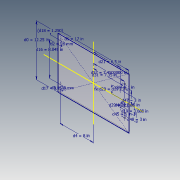
# Autodesk Inventor part: FLUGGER LOADING ACCESS DOOR
Saved by Autodesk Inventor 2020.3 (Build 243373000, 373)
## iProperties
RuleStatus: InUse
AfterDocSave0: file://Part Number Cleaner
Created: 2020-01-19
Material: ACRYLIC, CLEAR
Vendor: HHMI: JRC - ID&F
Document SubType Name: Modeling
Designer: arnoldj
Density: 0.66 g/cm^3
Appearance: Polycarbonate (Clear)
DESIGN DEPARTMENT: HHMI: JRC - ID&F
ALTERED ITEM PART NUMBER: N/A
ALTERED ITEM VENDOR: N/A
ALTERED ITEM DESCRIPTION: N/A
Author: arnoldj
Revision Number: 0
Autodesk Inventor part; units mm, degrees
ref_plane "YZ Plane" through (0, 0, 0) normal (1, 0, 0) x (0, 1, 0)
ref_plane "XZ Plane" through (0, 0, 0) normal (0, 1, 0) x (-1, 0, 0)
ref_plane "XY Plane" through (0, 0, 0) normal (0, 0, 1) x (1, 0, 0)
sketch "Sketch1" plane through (0, 0, 0) normal (0, 0, 1) x (1, 0, 0)
  line L0 (0, 217.805) -> (0, -217.805) projected
  line L1 (-302.26, 0) -> (302.26, 0) projected
  line L2 (215.9, -155.575) -> (-215.9, -155.575)
  line L3 (-215.9, -155.575) -> (-215.9, 155.575)
  line L4 (-215.9, 155.575) -> (215.9, 155.575)
  line L5 (215.9, 155.575) -> (215.9, -155.575)
  line L6 (215.9, -155.575) -> (-215.9, 155.575) construction
  line L7 (-215.9, -155.575) -> (215.9, 155.575) construction
  line L8 (186.69, -13.13) -> (186.69, -35.13) construction
  line L9 (189.23, 88.9) -> (189.23, 63.5) construction
  line L10 (189.23, -63.5) -> (189.23, -88.9) construction
  point P0 (0, 0)
  point P1 (-203.2, 123.818)
  point P2 (-203.2, 95.818)
  point P3 (-203.2, -108.525)
  point P4 (-203.2, -136.525)
  point P5 (165.1, 46.8376)
  point P6 (165.1, -46.8376)
  point P7 (186.69, -24.13)
  point P8 (189.23, -76.2)
  point P9 (189.23, 76.2)
  dimension "d0" = 311.15
  dimension "d1" = 431.8
  dimension "d2" = 28
  dimension "d3" = 28
  dimension "d4" = 203.2
  dimension "d16" = 204.343
  dimension "d17" = 19.05
  dimension "d18" = 31.757
  dimension "d19" = 93.6752
  dimension "d20" = 46.8376
  dimension "d21" = 165.1
  dimension "d29" = 22
  dimension "d31" = 186.69
  dimension "d44" = 25.4
  dimension "d45" = 25.4
  dimension "d46" = 24.13
  dimension "d47" = 76.2
  dimension "d48" = 76.2
  dimension "d57" = 189.23
  constraints: 18 end point, 8 vertical alignment, 5 midpoint, 3 vertical, 2 parallel, 1 horizontal, 1 perpendicular
  measures "d0" distance of L2.end L3.end
  measures "d1" distance of L3.end L4.end
  measures "d2" distance of point (-203.2, 95.818) point (-203.2, 123.818)
  measures "d3" distance of point (-203.2, -108.525) point (-203.2, -136.525)
  measures "d4" distance from line of point (-203.2, -136.525) L0
  measures "d16" distance of point (-203.2, -108.525) point (-203.2, 95.818)
  measures "d17" distance from line of point (-203.2, -136.525) L2
  measures "d18" distance from line of L4 point (-203.2, 123.818)
  measures "d19" distance of point (165.1, -46.838) point (165.1, 46.838)
  measures "d20" distance from line of point (165.1, 46.838) L1
  measures "d21" distance from line of L0 point (165.1, 46.838)
  measures "d29" distance of L8.end L8.start
  measures "d31" distance from line of L0 L8.start
  measures "d44" distance of L9.end L9.start
  measures "d45" distance of L10.start L10.end
  measures "d46" distance from line of L1 point (186.69, -24.13)
  measures "d47" distance from line of L1 point (189.23, 76.2)
  measures "d48" distance from line of point (189.23, -76.2) L1
  measures "d57" distance between parallel lines of L9 L0
extrude "Extrusion1" add sketch "Sketch1" against normal blind 6.35
hole "Hole1-Tap M5" at (-203.2, 123.818, 0) at (-203.2, 95.818, 0) at (-203.2, -108.525, 0) at (-203.2, -136.525, 0) direction (0, 0, -1) diameter 4.064 end through all
hole "Hole2-Tap M5" at (165.1, 46.8376, 0) at (165.1, -46.8376, 0) direction (0, 0, -1) diameter 4.064 end through all
hole "Hole3-Tap M4" at (186.69, -13.13, 0) at (186.69, -35.13, 0) direction (0, 0, -1) diameter 3.1242 end through all
fillet "Fillet1" radius 9.525 4 edges at (-215.9, 155.575, -3.175) (215.9, 155.575, -3.175) (215.9, -155.575, -3.175) (-215.9, -155.575, -3.175)
hole "Hole4 CSINK M4" at (189.23, -88.9, 0) at (189.23, 88.9, 0) at (189.23, 63.5, 0) at (189.23, -63.5, 0) direction (0, 0, -1) diameter 4.4958 end through all countersink diameter 9.398 countersink angle 90 clearance for "Flat Head Machine Screw" size "M4" standard "Ansi Metric M Profile"
equation "\"d20\" = 0.5 * d19"
body "Solid1"
